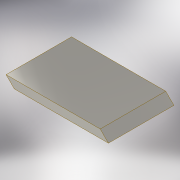
# Autodesk Inventor part: FieldOfView
Saved by Autodesk Inventor 2020 (Build 240168000, 168)
## iProperties
Created: 2020-07-31
Part Number: FieldOfView
Material: Titanium
Document SubType Name: Modeling
Designer: MicroscopyInnovation
Density: 4.51 g/cm^3
Appearance: Titanium
Author: MicroscopyInnovation
Autodesk Inventor part; units mm, degrees
ref_plane "YZ Plane" through (0, 0, 0) normal (1, 0, 0) x (0, 1, 0)
ref_plane "XZ Plane" through (0, 0, 0) normal (0, 1, 0) x (-1, 0, 0)
ref_plane "XY Plane" through (0, 0, 0) normal (0, 0, 1) x (1, 0, 0)
sketch "Sketch1" plane through (0, 0, 0) normal (0, 1, 0) x (-1, 0, 0)
  line L0 (-115, -80) -> (115, -80)
  line L1 (115, -80) -> (115, 80)
  line L2 (115, 80) -> (-115, 80)
  line L3 (-115, 80) -> (-115, -80)
  line L4 (-115, -80) -> (115, 80) construction
  line L5 (115, -80) -> (-115, 80) construction
  point P0 (0, 0)
  dimension "d0" = 230
  dimension "d1" = 160
  constraints: 12 end point, 2 midpoint, 2 parallel, 1 horizontal, 1 perpendicular
  measures "d0" distance of L2.end L1.end
  measures "d1" distance of L1.end L0.end
extrude "Extrusion1" add sketch "Sketch1" along normal blind 20
chamfer "Chamfer1" distance 20 angle 45 1 edges at (115, 20, 0)
sketch "Sketch2" plane through (-115, 0, -80) normal (-1, 0, 0) x (0, 0, 1)
  line L0 (0, 20) -> (160, 20) projected
  line L1 (0, 20) -> (160, 20)
  line L2 (160, 20) -> (160, 0)
  line L3 (160, 0) -> (0, 0)
  line L4 (0, 0) -> (0, 20)
  point P0 (80, 0)
  constraints: 8 end point, 2 parallel, 1 horizontal, 1 perpendicular
extrude "Extrusion2" add sketch "Sketch2" along normal blind 20
chamfer "Chamfer2" distance 20 angle 45 1 edges at (-135, 0, 0)
body "Solid1"
